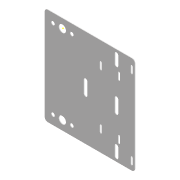
# Autodesk Inventor part: Part78
Saved by Autodesk Inventor 2020.5 (Build 245400000, 400)
## iProperties
Created: 2022-11-26
Part Number: Part78
Material: 一般
Document SubType Name: Modeling
Designer: Administrator
Density: 1 g/cm^3
Appearance: 既定
Author: Administrator
Autodesk Inventor part; units mm, degrees
ref_plane "YZ Plane" through (0, 0, 0) normal (1, 0, 0) x (0, 1, 0)
ref_plane "XZ Plane" through (0, 0, 0) normal (0, 1, 0) x (-1, 0, 0)
ref_plane "XY Plane" through (0, 0, 0) normal (0, 0, 1) x (1, 0, 0)
sketch "スケッチ1" plane through (0, 0, 0) normal (0, 0, 1) x (1, 0, 0)
  circle A0 centre (-15.5, 0) radius 2.5 projected
  circle A1 centre (15.5, 0) radius 2.5 projected
  circle A2 centre (0, 0) radius 11 projected
  line L0 (-15.1987, 13) -> (15.1987, 13) projected
  arc A3 (15.1987, -13) -> (15.1987, 13) centre (0, 0) ccw projected
  line L1 (15.1987, -13) -> (-15.1987, -13) projected
  arc A4 (-15.1987, 13) -> (-15.1987, -13) centre (0, 0) ccw projected
  circle A5 centre (-15.5, -130.182) radius 2.5 projected
  circle A6 centre (15.5, -130.182) radius 2.5 projected
  circle A7 centre (0, -130.182) radius 11 projected
  line L2 (-15.1987, -143.182) -> (15.1987, -143.182) projected
  arc A8 (-15.1987, -117.182) -> (-15.1987, -143.182) centre (0, -130.182) ccw projected
  line L3 (15.1987, -117.182) -> (-15.1987, -117.182) projected
  arc A9 (15.1987, -143.182) -> (15.1987, -117.182) centre (0, -130.182) ccw projected
  circle A10 centre (0, -130.182) radius 5 projected
  circle A11 centre (0, 0) radius 5 projected
  line L4 (-29, -33.3408) -> (-29, 14.909) projected
  line L5 (119, -145.0901) -> (-29, -145.0901) projected
  line L6 (-29, -63.3408) -> (-29, -33.3408)
  line L7 (119, 16.9081) -> (119, 16.909) projected
  line L8 (119, -145.0901) -> (119, 14.909)
  line L9 (119, 14.909) -> (112.6121, 14.909)
  line L10 (112.6121, 14.909) -> (112.6121, -145.0901)
  line L11 (112.6121, -145.0901) -> (119, -145.0901)
  circle A12 centre (0, -130.1819) radius 55
  circle A13 centre (0, 0.0009) radius 55
  line L12 (112.6121, -145.0901) -> (52.6121, -145.0901)
  line L13 (52.6121, -145.0901) -> (52.6121, 14.909)
  line L14 (52.6121, 14.909) -> (112.6121, 14.909)
  line L15 (112.6121, 14.909) -> (112.6121, -145.0901)
  line L16 (119, 14.909) -> (-29, 14.909) projected
  line L17 (119, 14.909) -> (119, -145.0901) projected
  line L18 (-29, -145.0901) -> (-29, -63.3408) projected
  arc A14 (-16.25, -63.3408) -> (-16.25, -33.3408) centre (-16.25, -48.3408) ccw projected
  circle A15 centre (-15.5, -130.1819) radius 3 projected
  circle A16 centre (-15.5, 0.0009) radius 3 projected
  circle A17 centre (0, 0.0009) radius 6 projected
  circle A18 centre (0, -130.1819) radius 6 projected
  circle A19 centre (15.5, -130.1819) radius 3 projected
  circle A20 centre (15.5, 0.0009) radius 3 projected
  circle A21 centre (14.75, -81.8408) radius 15 projected
  line L19 (-16.25, -33.3408) -> (-29, -33.3408) projected
  line L20 (-29, -63.3408) -> (-16.25, -63.3408) projected
  line L21 (88.1416, -96.2442) -> (88.1416, -36.2442) projected
  arc A22 (88.1416, -36.2442) -> (68.1416, -36.2442) centre (78.1416, -36.2442) ccw projected
  line L22 (68.1416, -36.2442) -> (68.1416, -96.2442) projected
  arc A23 (68.1416, -96.2442) -> (88.1416, -96.2442) centre (78.1416, -96.2442) ccw projected
  line L23 (91.6416, -106.2442) -> (91.6416, -116.2442) projected
  arc A24 (91.6416, -116.2442) -> (94.6416, -116.2442) centre (93.1416, -116.2442) ccw projected
  line L24 (94.6416, -116.2442) -> (94.6416, -106.2442) projected
  arc A25 (94.6416, -106.2442) -> (91.6416, -106.2442) centre (93.1416, -106.2442) ccw projected
  circle A26 centre (68.73, 9.909) radius 1.5 projected
  line L25 (41.1416, -74.7725) -> (41.1416, -54.7725) projected
  arc A27 (41.1416, -54.7725) -> (35.1416, -54.7725) centre (38.1416, -54.7725) ccw projected
  line L26 (35.1416, -54.7725) -> (35.1416, -74.7725) projected
  arc A28 (35.1416, -74.7725) -> (41.1416, -74.7725) centre (38.1416, -74.7725) ccw projected
  arc A29 (61.6416, -116.2442) -> (64.6416, -116.2442) centre (63.1416, -116.2442) ccw projected
  line L27 (64.6416, -116.2442) -> (64.6416, -106.2442) projected
  arc A30 (64.6416, -106.2442) -> (61.6416, -106.2442) centre (63.1416, -106.2442) ccw projected
  line L28 (61.6416, -106.2442) -> (61.6416, -116.2442) projected
  line L29 (112.5, -126.2399) -> (112.5, -136.2399) projected
  arc A31 (112.5, -136.2399) -> (115.5, -136.2399) centre (114, -136.2399) ccw projected
  line L30 (115.5, -136.2399) -> (115.5, -126.2399) projected
  arc A32 (115.5, -126.2399) -> (112.5, -126.2399) centre (114, -126.2399) ccw projected
  line L31 (91.6416, -16.2442) -> (91.6416, -26.2442) projected
  arc A33 (91.6416, -26.2442) -> (94.6416, -26.2442) centre (93.1416, -26.2442) ccw projected
  line L32 (94.6416, -26.2442) -> (94.6416, -16.2442) projected
  arc A34 (94.6416, -16.2442) -> (91.6416, -16.2442) centre (93.1416, -16.2442) ccw projected
  circle A35 centre (68.7299, -140.0901) radius 1.5 projected
  circle A36 centre (48.73, 9.909) radius 1.5 projected
  circle A37 centre (48.7299, -140.0901) radius 1.5 projected
  arc A38 (64.6416, -16.2442) -> (61.6416, -16.2442) centre (63.1416, -16.2442) ccw projected
  line L33 (61.6416, -16.2442) -> (61.6416, -26.2442) projected
  arc A39 (61.6416, -26.2442) -> (64.6416, -26.2442) centre (63.1416, -26.2442) ccw projected
  line L34 (64.6416, -26.2442) -> (64.6416, -16.2442) projected
  line L35 (112.5, 3.7592) -> (112.5, -6.2408) projected
  arc A40 (112.5, -6.2408) -> (115.5, -6.2408) centre (114, -6.2408) ccw projected
  line L36 (115.5, -6.2408) -> (115.5, 3.7592) projected
  arc A41 (115.5, 3.7592) -> (112.5, 3.7592) centre (114, 3.7592) ccw projected
  line L37 (92, -168.0931) -> (92, 36.9069) projected
  line L38 (86, 36.9069) -> (86, -168.0931) projected
  line L39 (203500644.9483, -137.7714) -> (203500644.9483, -122.7714) construction
  line L40 (203500647.9483, -137.7714) -> (203500647.9483, -122.7714)
  line L41 (203500641.9483, -122.7714) -> (203500641.9483, -137.7714)
  arc A42 (203500641.9483, -137.7714) -> (203500647.9483, -137.7714) centre (203500644.9483, -137.7714) ccw
  arc A43 (203500647.9483, -122.7714) -> (203500641.9483, -122.7714) centre (203500644.9483, -122.7714) ccw
  line L42 (89, 7.909) -> (89, -7.091) construction
  line L43 (92, 7.909) -> (92, -7.091)
  line L44 (86, -7.091) -> (86, 7.909)
  arc A44 (92, 7.909) -> (86, 7.909) centre (89, 7.909) ccw
  arc A45 (86, -7.091) -> (92, -7.091) centre (89, -7.091) ccw
  line L45 (87.3545, -74.7714) -> (87.3545, -54.7714) construction
  line L46 (90.3545, -74.7714) -> (90.3545, -54.7714)
  line L47 (84.3545, -54.7714) -> (84.3545, -74.7714)
  arc A46 (84.3545, -74.7714) -> (90.3545, -74.7714) centre (87.3545, -74.7714) ccw
  arc A47 (90.3545, -54.7714) -> (84.3545, -54.7714) centre (87.3545, -54.7714) ccw
  line L48 (-29, -145.0901) -> (-0.25, -145.0901)
  line L49 (-0.25, -145.0901) -> (-0.25, 14.909)
  line L50 (-0.25, 14.909) -> (-29, 14.909)
  line L51 (-29, 14.909) -> (-29, -145.0901)
  line L52 (19.75, -105.0901) -> (19.75, -25.0901)
  line L53 (19.75, -25.0901) -> (-20.25, -25.0901)
  line L54 (-20.25, -25.0901) -> (-20.25, -105.0901)
  line L55 (-20.25, -105.0901) -> (19.75, -105.0901)
  line L56 (19.75, -105.0901) -> (-20.25, -25.0901) construction
  line L57 (19.75, -25.0901) -> (-20.25, -105.0901) construction
  line L58 (19.75, -110.0901) -> (19.75, -20.0901)
  line L59 (19.75, -20.0901) -> (-20.25, -20.0901)
  line L60 (-20.25, -20.0901) -> (-20.25, -110.0901)
  line L61 (-20.25, -110.0901) -> (19.75, -110.0901)
  line L62 (19.75, -110.0901) -> (-20.25, -20.0901) construction
  line L63 (19.75, -20.0901) -> (-20.25, -110.0901) construction
  circle A48 centre (19.75, -110.0901) radius 1.5
  circle A49 centre (19.75, -20.0901) radius 1.5
  circle A50 centre (-20.25, -20.0901) radius 1.5
  circle A51 centre (-20.25, -110.0901) radius 1.5
  line L64 (88.9576, -138.0901) -> (88.9576, -123.0901) construction
  line L65 (91.9576, -138.0901) -> (91.9576, -123.0901)
  line L66 (85.9576, -123.0901) -> (85.9576, -138.0901)
  arc A52 (85.9576, -138.0901) -> (91.9576, -138.0901) centre (88.9576, -138.0901) ccw
  arc A53 (91.9576, -123.0901) -> (85.9576, -123.0901) centre (88.9576, -123.0901) ccw
  point P0 (0, 0)
  point P1 (203500644.9483, -130.2714)
  point P2 (89, 0.409)
  point P3 (92, 7.909)
  point P4 (92, -7.091)
  point P5 (86, -7.094)
  point P6 (86, 7.9123)
  point P7 (92, -138.091)
  point P8 (86, -140.5013)
  point P9 (86, -123.0862)
  point P10 (92, -123.0898)
  point P11 (87.3545, -64.7714)
  point P12 (86, -7.0941)
  point P13 (86, 7.909)
  point P14 (92, -55.0901)
  point P15 (92, -75.0901)
  point P16 (86, -77.4482)
  point P17 (86, -52.0946)
  point P18 (92, -138.0901)
  point P19 (86, -138.0901)
  point P20 (86, -120.6788)
  point P21 (92, -123.0901)
  point P22 (114.2151, 14.909)
  point P23 (114.2151, 14.909)
  point P24 (-0.25, -65.0901)
  point P25 (86, -7.0941)
  point P26 (86, -7.091)
  point P27 (88.9576, -130.5901)
  point P28 (86, -138.5928)
  point P29 (86, -122.5873)
  dimension "d7" = 15
  dimension "d8" = 6
  dimension "d2" = 110
  dimension "d3" = 110
  dimension "d4" = 60
  dimension "d5" = 159.9991
  dimension "d9" = 7
  dimension "d10" = 7
  dimension "d11" = 15
  dimension "d12" = 6
  dimension "d13" = 48
  dimension "d14" = 20
  dimension "d17" = 80
  dimension "d18" = 40
  dimension "d19" = 159.9991
  dimension "d20" = 80
  dimension "d21" = 90
  dimension "d22" = 40
  dimension "d23" = 3
  dimension "d24" = 3
  dimension "d25" = 3
  dimension "d26" = 3
  dimension "d27" = 15
  dimension "d28" = 6
  dimension "d29" = 7
  constraints: 74 end point, 14 parallel, 12 centre point, 12 point on circle, 12 tangent, 7 midpoint, 5 perpendicular, 4 coincident, 3 point on line, 3 vertical, 1 horizontal, 3 other
  measures "d2" diameter of A12
  measures "d3" diameter of A13
  measures "d4" distance of L10.end L12.end
  measures "d5" distance between parallel lines of L14 L12
  measures "d10" distance from line of L16 L42.start
  measures "d11" distance of L42.end L42.start
  measures "d12" diameter of A47
  measures "d14" distance of L45.end L45.start
  measures "d17" distance of L52.start L52.end
  measures "d18" distance of L53.end L52.end
  measures "d19" distance between parallel lines of L16 L5
  measures "d20" distance from line of L5 point (-0.25, -65.09)
  measures "d21" distance of L58.start L58.end
  measures "d22" distance of L59.end L58.end
  measures "d23" diameter of A48
  measures "d24" diameter of A49
  measures "d25" diameter of A50
  measures "d26" diameter of A51
  measures "d27" distance of L64.start L64.end
  measures "d28" diameter of A53
  measures "d29" distance from line of L12 L64.start
extrude "押し出し1" add sketch "スケッチ1" along normal blind 1 contours A2 L49 A17 | A2 L49 L0 A3 L1 | L49 A17 A2 | A2 L49 L1 A4 L0 | L49 L16 L13 A13 L52 L58 A49 L59 L1 A3 L0 | L0 A4 L1 L49 L59 A50 L60 L54 L19 L4 L16 | L59 A49 L58 L53 L49 | L49 L53 L60 A50 L59 | L14 A13 L13 | L53 L52 A13 L49 | L49 A13 A14 L19 L54 L53 | L13 A12 A21 L52 A13 | A13 L14 L38 A22 L22 A23 A53 L66 A52 L5 A12 L13 | L19 L54 A13 L6 | L49 A12 L54 L20 A14 A13 | A13 L52 A21 A12 L49 | L13 L5 L49 L2 A9 L3 L61 A48 L58 L52 A21 A12 | A12 L5 L13 | A13 L54 L20 L6 | L14 L37 A44 L38 | L19 A14 A13 L54 | A14 L20 L54 A13 | L49 L55 L54 A12 | A12 A21 L49 | L52 A12 A21 | A21 A12 L52 | A21 L52 A12 | L20 L54 A12 L18 | L14 L10 A41 L35 A40 A32 L29 A31 L5 L37 A24 L24 A25 A33 L32 A34 | A12 L52 A21 | L54 L60 A51 L61 L49 L3 A8 L2 L5 L18 A12 | A21 L52 L55 L49 | L9 L8 L5 L10 A31 L30 A32 A40 L36 A41 | A45 L37 A34 L31 A33 A25 L23 A24 L5 L38 A52 L65 A53 A23 L21 A46 L46 A47 A22 | L55 L49 L61 A51 L60 | L55 L58 A48 L61 L49 | L49 A7 L3 A9 L2 | L2 A8 L3 L49 A7 | L38 A47 L47 A46 A23 L22 A22 | A22 L21 A47 L38 | A52 L66 A53 L38 | L49 A18 A7 | A7 L49 A18 | A46 L21 A23 L38 | A26 | A35 | A36 | A37
sketch "スケッチ2" plane through (0, 0, 0) normal (0, 0, -1) x (-1, 0, 0)
  point P0 (0, 0)
fillet "フィレット1" radius 5 4 edges at (-29, -145.0901, 0.5) (-29, 14.909, 0.5) (119, -145.0901, 0.5) (119, 14.909, 0.5)
